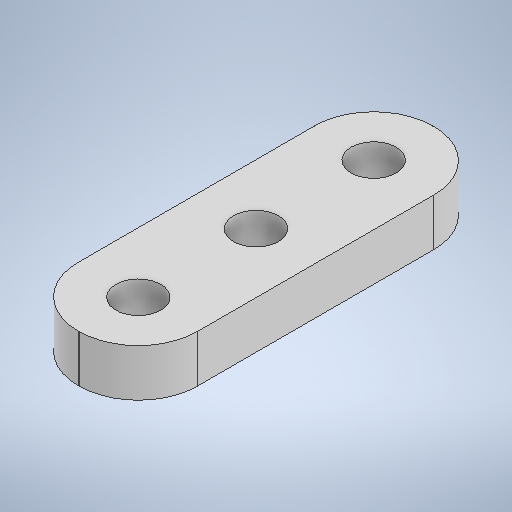
# Autodesk Inventor part: Part4
Saved by Autodesk Inventor 2025.3 (Build 293356000, 356)
## iProperties
Created: 2025-07-14
Part Number: Part4
Material: Generic
Document SubType Name: Modeling
Designer: steve
Density: 1 g/cm^3
Appearance: Default
Author: steve
Autodesk Inventor part; units mm, degrees
ref_plane "YZ Plane" through (0, 0, 0) normal (1, 0, 0) x (0, 1, 0)
ref_plane "XZ Plane" through (0, 0, 0) normal (0, 1, 0) x (-1, 0, 0)
ref_plane "XY Plane" through (0, 0, 0) normal (0, 0, 1) x (1, 0, 0)
sketch "Sketch1" plane through (0, 0, 0) normal (0, 1, 0) x (-1, 0, 0)
  line L0 (-0.025, -7.5) -> (0.025, -7.5)
  line L1 (2.525, -5) -> (2.525, 5)
  line L2 (0.025, 7.5) -> (-0.025, 7.5)
  line L3 (-2.525, 5) -> (-2.525, -5)
  line L4 (-2.525, -7.5) -> (2.525, 7.5) construction
  line L5 (2.525, -7.5) -> (-2.525, 7.5) construction
  arc A0 (2.525, 5) -> (0.025, 7.5) centre (0.025, 5) ccw
  arc A1 (-0.025, 7.5) -> (-2.525, 5) centre (-0.025, 5) ccw
  arc A2 (-2.525, -5) -> (-0.025, -7.5) centre (-0.025, -5) ccw
  arc A3 (0.025, -7.5) -> (2.525, -5) centre (0.025, -5) ccw
  circle A4 centre (0, 0) radius 0.95
  circle A5 centre (-0.025, 5) radius 0.95
  circle A6 centre (0.025, -5) radius 0.95
  dimension "d0" = 5.05
  dimension "d1" = 15
  dimension "d2" = 2.5
  dimension "d3" = 1.9
  dimension "d4" = 1.9
  dimension "d5" = 1.9
  constraints: 12 end point, 8 point on circle, 8 point on line, 8 tangent, 7 centre point, 3 coincident, 3 equal radius, 2 midpoint, 2 parallel, 1 horizontal, 1 perpendicular
  measures "d0" distance of L5.end L4.end
  measures "d1" distance of L4.end L5.start
  measures "d2" radius of A0
  measures "d3" diameter of A4
  measures "d4" diameter of A5
  measures "d5" diameter of A6
extrude "Extrusion1" add sketch "Sketch1" along normal blind 2
body "Solid1"
